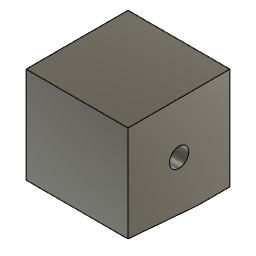
locking_seal_bracket v1 (Autodesk Fusion 360 design; units mm, degrees)
Autodesk Fusion 360 part; units mm, degrees
sketch "Sketch1" plane through (0, 0, 0) normal (0, 0, 1) x (1, 0, 0)
  line L0 (0, 0) -> (17.5, 0)
  line L1 (17.5, 0) -> (17.5, 17.5)
  line L2 (17.5, 17.5) -> (0, 17.5)
  line L3 (0, 17.5) -> (0, 0)
  dimension "d1" = 17.5
  dimension "d2" = 17.5
  constraint horizontal L0
  constraint vertical L1
  constraint horizontal L2
  constraint vertical L3
  constraint coincident L0.start L3.end
  measures "d1" distance of L0.start L0.end
  measures "d2" distance of L0.start L2.end
extrude "Extrude1" add sketch "Sketch1" along normal blind 17.5
sketch "Sketch2" plane through (0, 0, 0) normal (-1, 0, 0) x (0, -1, 0)
  line L0 (-17.5, 0) -> (0, 0)
  line L1 (0, 0) -> (0, 17.5)
  line L2 (0, 17.5) -> (-17.5, 17.5)
  line L3 (-17.5, 17.5) -> (-17.5, 0)
  circle A0 centre (-8.7787, 8.7562) radius 8.7563
  circle A1 centre (-8.7787, 8.7562) radius 1.65
  dimension "d5" = 3.3
  constraint concentric A0 A1
  measures "d5" diameter of A1
extrude "Extrude2" cut sketch "Sketch2" against normal blind 33 contours A1
chamfer "Chamfer1" distance 1 distance2 12 1 edges at (8.75, 0, 0) measured on face at (5.8333, 0, 5.8333)
